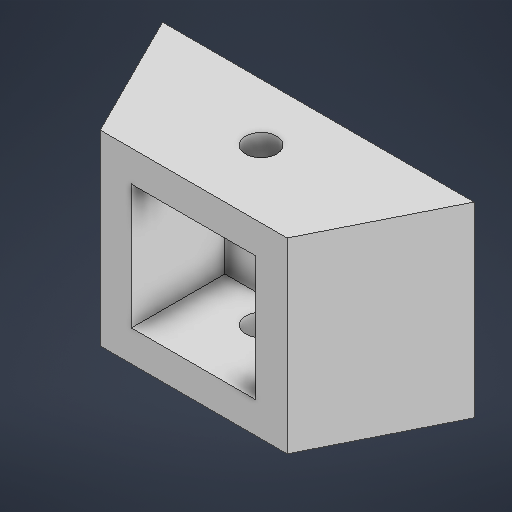
# Autodesk Inventor part: base de soporte
Saved by Autodesk Inventor 2026.1 (Build 301233020, 233B)
## iProperties
Created: 2025-10-30
Part Number: base de soporte
Material: Generic
Document SubType Name: Sheet Metal
Designer: Tito Luyo Murata
Density: 1 g/cm^3
Sheet Metal Rule: Default_mm
Appearance: Default
Author: Tito Luyo Murata
Autodesk Inventor part; units mm, degrees
ref_plane "YZ Plane" through (0, 0, 0) normal (1, 0, 0) x (0, 1, 0)
ref_plane "XZ Plane" through (0, 0, 0) normal (0, 1, 0) x (-1, 0, 0)
ref_plane "XY Plane" through (0, 0, 0) normal (0, 0, 1) x (1, 0, 0)
sketch "Sketch1" plane through (0, 0, 0) normal (0, 0, 1) x (1, 0, 0)
  line L0 (0, 0) -> (30, 0)
  line L1 (30, 0) -> (30, -30)
  line L2 (30, -30) -> (0, -30)
  line L3 (0, -30) -> (0, 0)
  line L4 (0, 0) -> (5, 0)
  line L5 (5, -5.8022) -> (25, -5.8022)
  line L6 (25, -5.8022) -> (25, -25.8022)
  line L7 (25, -25.8022) -> (5, -25.8022)
  line L8 (5, -25.8022) -> (5, -5.8022)
  dimension "d0" = 30
  dimension "d1" = 30
  dimension "d6" = 20
  dimension "d7" = 20
  constraints: 18 end point, 4 parallel, 2 horizontal, 2 perpendicular
  measures "d0" distance of L1.end L2.end
  measures "d1" distance of L0.end L1.end
  measures "d6" distance of L6.end L7.end
  measures "d7" distance of L5.end L6.end
extrude "Extrusion1" add sketch "Sketch1" along normal blind 20 contours L0 L1 L2 L3 | L5 L6 L7 L8
sketch "Sketch2" plane through (0, 0, 20) normal (0, 0, 1) x (1, 0, 0)
  line L0 (30, 0) -> (0, 0) projected
  line L1 (0, 0) -> (5, 0)
  line L2 (5, -5) -> (25, -5)
  line L3 (25, -5) -> (25, -25)
  line L4 (25, -25) -> (5, -25)
  line L5 (5, -25) -> (5, -5)
  dimension "d8" = 5
  constraints: 10 end point, 2 parallel, 1 horizontal, 1 perpendicular, 1 point on line
  measures "d8" distance of L0.end L1.end
extrude "Extrusion2" cut sketch "Sketch2" against normal blind 15
sketch "Sketch3" plane through (0, -30, 0) normal (0, -1, 0) x (1, 0, 0)
  line L0 (0, 0) -> (-10, 0)
  line L1 (0, 0) -> (0, 20) projected
  line L2 (-10, 0) -> (0, 20)
  dimension "d14" = 10
  constraints: 4 end point, 1 horizontal
  measures "d14" distance of L0.start L0.end
extrude "Extrusion3" add sketch "Sketch3" against normal blind 30
sketch "Sketch4" plane through (30, -30, 0) normal (0, -1, 0) x (1, 0, 0)
  line L0 (-40, 0) -> (0, 0) projected
  line L1 (0, 0) -> (10, 0)
  line L2 (0, 0) -> (0, 20) projected
  line L3 (10, 0) -> (0, 20)
  point P0 (-30, 0)
  dimension "d17" = 10
  constraints: 4 end point, 1 horizontal
  measures "d17" distance of L0.end L1.end
extrude "Extrusion4" add sketch "Sketch4" against normal blind 30
sketch "Sketch5" plane through (-10, -30, 0) normal (0, -1, 0) x (1, 0, 0)
  line L0 (10, 9.1728) -> (40, 9.1728)
  line L1 (15, 20) -> (35, 20) projected
  line L2 (25, 20) -> (25, 9.1728)
  circle A0 centre (25, 9.1728) radius 2.5
  point P0 (10, 0)
  dimension "d21" = 5
  constraints: 4 end point, 2 midpoint, 1 centre point, 1 coincident, 1 horizontal
  measures "d21" diameter of A0
extrude "Extrusion5" cut sketch "Sketch5" against normal blind 30
equation "\"BendRadius\" = Thickness"
equation "\"BendReliefWidth\" = Thickness"
equation "\"BendReliefDepth\" = 0.5 * Thickness"
equation "\"CornerReliefSize\" = 4 * Thickness"
equation "\"MinimumRemnant\" = 2 * Thickness"
equation "\"TransitionRadius\" = BendRadius"
equation "\"JacobiRadiusSize\" = BendRadius"
equation "\"GapSize\" = Thickness"
equation "\"Thickness\" = 0.5"
body "Solid1"
